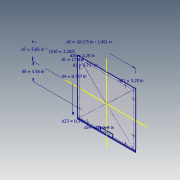
# Autodesk Inventor part: FLUGGER SIDE COVER
Saved by Autodesk Inventor 2020.3 (Build 243373000, 373)
## iProperties
RuleStatus: InUse
AfterDocSave0: file://Part Number Cleaner
Created: 2020-01-03
Material: ACRYLIC, CLEAR
Vendor: HHMI: JRC - ID&F
Document SubType Name: Modeling
Designer: arnoldj
Density: 0.66 g/cm^3
Appearance: Polycarbonate (Clear)
DESIGN DEPARTMENT: HHMI: JRC - ID&F
ALTERED ITEM PART NUMBER: N/A
ALTERED ITEM VENDOR: N/A
ALTERED ITEM DESCRIPTION: N/A
Author: arnoldj
Revision Number: 0
Autodesk Inventor part; units mm, degrees
ref_plane "YZ Plane" through (0, 0, 0) normal (1, 0, 0) x (0, 1, 0)
ref_plane "XZ Plane" through (0, 0, 0) normal (0, 1, 0) x (-1, 0, 0)
ref_plane "XY Plane" through (0, 0, 0) normal (0, 0, 1) x (1, 0, 0)
sketch "Sketch1" plane through (0, 0, 0) normal (0, 0, 1) x (1, 0, 0)
  line L0 (0, 316.484) -> (0, -316.484) projected
  line L1 (-334.6907, 0) -> (334.6907, 0) projected
  line L2 (239.0648, -226.06) -> (-239.0648, -226.06)
  line L3 (-239.0648, -226.06) -> (-239.0648, 226.06)
  line L4 (-239.0648, 226.06) -> (239.0648, 226.06)
  line L5 (239.0648, 226.06) -> (239.0648, -226.06)
  line L6 (239.0648, -226.06) -> (-239.0648, 226.06) construction
  line L7 (-239.0648, -226.06) -> (239.0648, 226.06) construction
  line L8 (220.345, -207.3402) -> (-220.345, -207.3402) construction
  line L9 (-220.345, -207.3402) -> (-220.345, 207.3402) construction
  line L10 (-220.345, 207.3402) -> (220.345, 207.3402) construction
  line L11 (220.345, 207.3402) -> (220.345, -207.3402) construction
  line L12 (220.345, -207.3402) -> (-220.345, 207.3402) construction
  line L13 (-220.345, -207.3402) -> (220.345, 207.3402) construction
  line L14 (-239.0648, -218.44) -> (239.0648, -218.44)
  line L15 (50.8, -191.06) -> (-50.8, -191.06)
  line L16 (-50.8, -191.06) -> (-50.8, -218.44)
  line L17 (-50.8, -218.44) -> (50.8, -218.44)
  line L18 (50.8, -218.44) -> (50.8, -191.06)
  line L19 (50.8, -191.06) -> (-50.8, -218.44) construction
  line L20 (-50.8, -191.06) -> (50.8, -218.44) construction
  point P0 (0, 0)
  point P1 (-156.5148, 207.3402)
  point P2 (0, 207.3402)
  point P3 (156.5148, 207.3402)
  point P4 (-156.5148, -207.3402)
  point P5 (0, -207.3402)
  point P6 (156.5148, -207.3402)
  point P7 (-220.345, 143.51)
  point P8 (-220.345, -143.51)
  point P9 (220.345, 143.51)
  point P10 (220.345, -117.0967)
  point P11 (-220.345, 0)
  point P12 (0, -218.44)
  point P13 (0, -226.06)
  point P14 (0, -204.75)
  point P15 (50.8, -218.44)
  dimension "d0" = 478.1296
  dimension "d1" = 452.12
  dimension "d3" = 18.7198
  dimension "d4" = 18.7198
  dimension "d7" = 143.51
  dimension "d8" = 143.51
  dimension "d10" = 82.55
  dimension "d20" = 82.55
  dimension "d21" = 82.55
  dimension "d23" = 7.62
  dimension "d24" = 35
  dimension "d25" = 101.6
  constraints: 38 end point, 12 point on line, 9 midpoint, 6 parallel, 4 coincident, 4 perpendicular, 3 horizontal, 2 vertical alignment, 1 horizontal alignment
  measures "d0" distance of L3.end L4.end
  measures "d1" distance of L2.end L3.end
  measures "d3" distance between parallel lines of L10 L4
  measures "d4" distance between parallel lines of L9 L3
  measures "d7" distance from line of L1 point (-220.345, 143.51)
  measures "d8" distance from line of point (-220.345, -143.51) L1
  measures "d10" distance from line of point (-220.345, 143.51) L4
  measures "d20" distance from line of point (-156.515, 207.34) L3
  measures "d21" distance from line of L5 point (156.515, 207.34)
  measures "d23" distance between parallel lines of L14 L2
  measures "d24" distance between parallel lines of L2 L15
  measures "d25" distance of L15.start L15.end
extrude "Extrusion1" add sketch "Sketch1" against normal blind 4.4958 contours L4 L5 L1 L0 | L0 L1 L3 L4 | L1 L5 L14 L18 L15 L0 | L0 L15 L16 L14 L3 L1
hole "Hole1" at (-156.5148, 207.3402, 0) at (156.5148, 207.3402, 0) at (-156.5148, -207.3402, 0) at (156.5148, -207.3402, 0) at (220.345, 143.51, 0) at (220.345, -117.0967, 0) at (-220.345, 143.51, 0) at (-220.345, -143.51, 0) direction (0, 0, -1) diameter 8.255 end through all
fillet "Fillet1" radius 9.525 2 edges at (-239.0648, 226.06, -2.2479) (239.0648, 226.06, -2.2479)
fillet "Fillet2" radius 9.525 2 edges at (-239.0648, -218.44, -2.2479) (239.0648, -218.44, -2.2479)
fillet "Fillet3" radius 3.175 4 edges at (50.8, -191.06, -2.2479) (50.8, -218.44, -2.2479) (-50.8, -191.06, -2.2479) (-50.8, -218.44, -2.2479)
body "Solid1"
